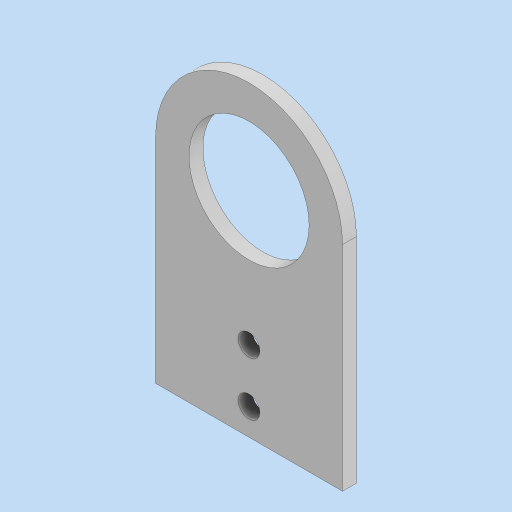
# Autodesk Inventor part: ArmPlateBase
Saved by Autodesk Inventor 2024 (Build 280153000, 153)
## iProperties
Created: 2024-01-11
Part Number: ArmPlateBase
Material: Generic
Document SubType Name: Modeling
Designer: megan
Density: 1 g/cm^3
Appearance: Default
Author: megan
Autodesk Inventor part; units mm, degrees
ref_plane "YZ Plane" through (0, 0, 0) normal (1, 0, 0) x (0, 1, 0)
ref_plane "XZ Plane" through (0, 0, 0) normal (0, 1, 0) x (-1, 0, 0)
ref_plane "XY Plane" through (0, 0, 0) normal (0, 0, 1) x (1, 0, 0)
sketch "Sketch1" plane through (0, 0, 0) normal (0, 0, 1) x (1, 0, 0)
  arc A0 (22.225, 0) -> (-22.225, 0) centre (0, 0) ccw
  circle A1 centre (0, 0) radius 14.2875
  line L0 (-22.225, -50.8) -> (22.225, -50.8)
  line L1 (22.225, -50.8) -> (22.225, 0)
  line L2 (-22.225, 0) -> (-22.225, -50.8)
  line L3 (0, -65.405) -> (0, 36.83) projected
  circle A2 centre (0, -31.75) radius 2.5781
  circle A3 centre (0, -44.45) radius 2.5781
  dimension "d0" = 44.45
  dimension "d1" = 28.575
  dimension "d3" = 5.1562
  dimension "d4" = 5.1562
  dimension "d5" = 12.7
  dimension "d6" = 6.35
  dimension "d7" = 31.75
  constraints: 6 end point, 4 centre point, 3 parallel, 2 coincident, 2 point on circle, 2 point on line, 1 perpendicular, 1 tangent
  measures "d0" diameter of A0
  measures "d1" diameter of A1
  measures "d3" diameter of A2
  measures "d4" diameter of A3
  measures "d5" distance of A3.centre A2.centre
  measures "d6" distance from line of L0 A3.centre
  measures "d7" distance of A2.centre A0.centre
extrude "Extrusion1" add sketch "Sketch1" along normal blind 3.302 contours L1 L0 L3 A3 A2 A1 A0 | L3 A1 A2 A3 L0 L2 A0
body "Solid1"
